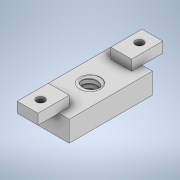
# Autodesk Inventor part: hires mount for beamsplitter test
Saved by Autodesk Inventor 2022 (Build 260153000, 153)
## iProperties
Created: 2022-07-06
Part Number: hires mount for beamsplitter test
Material: Generic
Document SubType Name: Modeling
Designer: Eli
Density: 1 g/cm^3
Appearance: Default
Author: Eli
Autodesk Inventor part; units mm, degrees
sketch "Sketch1" plane through (0, 0, 0) normal (0, 1, 0) x (-1, 0, 0)
  line L0 (0, 0) -> (-12.7, 0)
  line L1 (-12.7, 0) -> (-12.7, -25.4)
  line L2 (-12.7, -25.4) -> (0, -25.4)
  line L3 (0, -25.4) -> (0, 0)
  line L4 (-3.175, -25.4) -> (-9.525, -25.4)
  dimension "d1" = 12.7
  dimension "d82" = 25.4
  constraints: 10 end point, 2 horizontal, 2 parallel, 1 perpendicular, 1 point on line
  measures "d1" distance of L0.start L0.end
  measures "d82" distance between parallel lines of L0 L4
extrude "Extrusion1" add sketch "Sketch1" along normal blind 6.35
sketch "Sketch2" plane through (0, 0, 0) normal (0, -1, 0) x (1, 0, 0)
  line L0 (0, -25.4) -> (0, 0) projected
  line L1 (0, -12.7) -> (12.7, -12.7) construction
  line L2 (12.7, 0) -> (12.7, -25.4) projected
  line L3 (0, 0) -> (12.7, 0) projected
  line L4 (6.35, 0) -> (6.35, -25.4) construction
  line L5 (12.7, -25.4) -> (0, -25.4) projected
  point P0 (6.35, -12.7)
  constraints: 5 midpoint, 4 end point
hole "Hole1" at (6.35, 0, -12.7) direction (0, 1, 0) diameter 6.35 depth 6.35
thread "Thread1" size "1/4-20 UNC" class "2B" standard "ANSI Unified Screw Threads" full length
ref_plane "Work Plane3" through (3.175, 6.35, -3.175) normal (0, 0, 1) x (1, 0, 0)
sketch "Sketch7" plane through (3.175, 6.35, -3.175) normal (0, 0, 1) x (1, 0, 0)
  line L0 (0, 3.175) -> (6.35, 3.175) projected
  line L1 (6.35, 0) -> (6.35, 3.175) projected
  line L2 (0, 3.175) -> (6.35, 3.175)
  line L3 (6.35, 3.175) -> (6.35, 0)
  line L4 (6.35, 0) -> (0, 0)
  line L5 (0, 0) -> (0, 3.175)
  point P0 (-3.175, -6.35)
  dimension "d32" = 3.175
  constraints: 8 end point, 2 parallel, 1 horizontal, 1 perpendicular, 1 point on line
  measures "d32" distance of L4.end L0.start
extrude "Extrusion4" add sketch "Sketch7" along normal blind 9.525
ref_plane "Work Plane4" through (0, 9.525, 0) normal (0, 1, 0) x (1, 0, 0)
sketch "Sketch12" plane through (6.35, 0, -12.7) normal (-1, 0, 0) x (0, 0, 1)
  line L0 (3.175, 0) -> (3.175, 6.35)
  line L1 (3.175, 6.35) -> (2.2333, 6.35)
  line L2 (2.2333, 6.35) -> (2.2333, 0)
  line L3 (2.2333, 0) -> (3.175, 0)
  line L4 (0, -1.27) -> (0, 7.62) projected
  constraints: 8 end point
revolve "Revolution2" add sketch "Sketch12" angle 360 about axis through (6.35, 0, -12.7) along (0, 1, 0) separate body
sketch "Sketch8" plane through (0, 9.525, 0) normal (0, 1, 0) x (1, 0, 0)
  line L0 (12.7, 0) -> (12.7, 25.4) construction
  line L1 (12.7, 12.7) -> (0, 12.7) construction
  line L2 (6.35, 12.7) -> (6.35, -6.35) construction
  line L3 (3.175, -6.35) -> (9.525, -6.35) construction
  point P0 (0, 0)
  point P1 (6.35, -2.3812)
  dimension "d35" = 15.0813
  constraints: 4 end point, 3 midpoint, 1 horizontal, 1 point on line, 1 vertical
  measures "d35" distance from line of L1 point (6.35, -2.381)
hole "Hole3" at (6.35, 9.525, 2.3812) direction (0, -1, 0) diameter 2.54 depth 3.175 bodies 1
ref_plane "Work Plane2" through (12.7, 6.35, -12.7) normal (0, 0, -1) x (-1, 0, 0)
sketch "Sketch11" plane through (6.35, 0, -9.525) normal (1, 0, 0) x (0, 1, 0)
  line L0 (-0.7409, -0.0644) -> (-0.6351, -0.0644) construction
  line L1 (0.1057, -0.8776) -> (-0.0001, -1.0809) construction
  line L2 (-1.2701, -1.0809) -> (-1.3759, -0.8776) construction
  line L3 (-0.5293, -0.0644) -> (-0.6351, 0.1389) construction
  line L4 (-0.6351, 0.1389) -> (-0.7409, -0.0644) construction
  line L5 (-1.2701, -1.0809) -> (-1.1643, -0.8776) construction
  line L6 (-0.5293, -0.0644) -> (-0.1059, -0.8776)
  line L7 (-1.3759, -0.8776) -> (-1.1643, -0.8776) construction
  arc A0 (-1.3759, -0.8776) -> (-1.2701, -0.9418) centre (-1.2701, -0.8225) ccw construction
  line L8 (0.1057, -0.8776) -> (-0.1059, -0.8776) construction
  line L9 (-1.2701, -1.0809) -> (-1.2701, -0.8776) construction
  line L10 (-0.0001, -1.0809) -> (-0.0001, -0.8776) construction
  line L11 (-0.6351, 0.1389) -> (-0.6351, -0.0002) construction
  line L12 (-1.2701, -0.9418) -> (-0.0001, -0.9418)
  arc A1 (-1.2701, -0.9418) -> (-1.1643, -0.8776) centre (-1.2701, -0.8225) ccw
  line L13 (-0.1059, -0.8776) -> (-0.0001, -1.0809) construction
  line L14 (-1.1643, -0.8776) -> (-0.7409, -0.0644)
  line L15 (-0.0001, -0.0002) -> (-0.0001, 0.0177)
  line L16 (-0.0001, 0.0177) -> (-0.0001, -0.0002)
  line L17 (-0.0001, -0.0002) -> (0.0334, -0.0002)
  arc A2 (-0.1059, -0.8776) -> (-0.0001, -0.9418) centre (-0.0001, -0.8225) ccw
  arc A3 (-0.0001, -0.9418) -> (0.1057, -0.8776) centre (-0.0001, -0.8225) ccw construction
  arc A4 (-0.6351, -0.0002) -> (-0.7409, -0.0644) centre (-0.6351, -0.1195) ccw
  arc A5 (-0.5293, -0.0644) -> (-0.6351, -0.0002) centre (-0.6351, -0.1195) ccw
  line L18 (-0.6351, -0.0002) -> (-0.6351, -0.0644) construction
  line L19 (-0.6351, -0.0644) -> (-0.5293, -0.0644) construction
  dimension "d61" = 55
  dimension "d62" = 0.2033
  dimension "d63" = 0.2033
  dimension "Sketch11_ThreadOffset" = 0
  dimension "Sketch11_MajorRadius" = 0.9417
  dimension "d66" = 1.27
  dimension "Sketch11_MinorRadius" = 0
  constraints: 40 end point, 12 point on circle, 10 parallel, 8 tangent, 6 centre point, 6 collinear, 2 midpoint, 2 point on line, 1 horizontal, 1 perpendicular, 3 other
  measures "d61" angle of L6 L14
  measures "d62" distance of L3.end L0.end
  measures "d63" distance of L1.end L10.end
  measures "Sketch11_ThreadOffset" distance between parallel lines of L15 L10
  measures "Sketch11_MajorRadius" distance from line of L12 L15.start
  measures "d66" distance from line of L1.end L9
  measures "Sketch11_MinorRadius" distance edge to line of A5 L17
coil "Coil2" sketch "Sketch11" operation cut axis through (6.35, 0, -12.7) along (0, 1, 0) pitch 1.2713 turns 6.993007 hand right bodies 2
ref_plane "Work Plane5" through (0, 0, -12.7) normal (0, 0, 1) x (1, 0, 0)
mirror "Mirror3" about plane through (0, 0, -12.7) normal (0, 0, 1) of "Extrusion4", "Hole3" bodies 1
equation "\"d61\" = d68"
equation "\"d62\" = 0.160083 * Sketch11_Pitch"
equation "\"d63\" = 0.160083 * Sketch11_Pitch"
equation "\"d66\" = Sketch11_Pitch"
equation "\"d50\" = 55deg"
equation "\"Sketch9_Pitch\" = 1.27"
equation "\"d68\" = 55deg"
equation "\"Sketch11_Pitch\" = 1.27"
body "Solid1"
body "Solid3"
